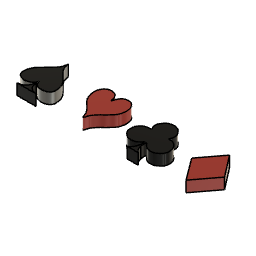
extrusion (Autodesk Fusion 360 design; units mm, degrees)
Autodesk Fusion 360 part; units mm, degrees
note: some values were not read from the file. Set by a fixed rule: which sketch regions a step uses.
sketch "Sketch1" plane through (0, 0, 0) normal (0, 0, 1) x (1, 0, 0)
  line L0 (72.8939, 22.1352) -> (57.9762, 2.4076)
  line L1 (57.9762, 2.4076) -> (72.8939, -17.6718)
  line L2 (72.8939, -17.6718) -> (88.0776, 2.4076)
  line L3 (88.0776, 2.4076) -> (72.8939, 22.1352)
  spline S0 degree 5 poles (16.5531, 7.024) (16.5732, 7.0699) (16.5975, 7.1734) (16.5852, 7.3637) (16.4741, 7.6811) (16.2192, 8.1458) (15.9092, 8.6303) (15.609, 9.0883) (15.3735, 9.4853) (15.2319, 9.8114) (15.1766, 10.0886) (15.1804, 10.3537) (15.2084, 10.645) (15.2326, 10.9866) (15.2428, 11.3775) (15.2401, 11.8016) (15.2341, 12.2351) (15.2374, 12.6541) (15.2624, 13.0428) (15.3167, 13.4004) (15.4043, 13.7352) (15.5255, 14.0605) (15.6783, 14.3894) (15.858, 14.7294) (16.0583, 15.081) (16.2727, 15.44) (16.4956, 15.8002) (16.7233, 16.1555) (16.9554, 16.5019) (17.1957, 16.8395) (17.4501, 17.1706) (17.7254, 17.4981) (18.0274, 17.8239) (18.3599, 18.1476) (18.7223, 18.4645) (19.1106, 18.7666) (19.5188, 19.0446) (19.9396, 19.2893) (20.3664, 19.4939) (20.7937, 19.6552) (21.2193, 19.7758) (21.6435, 19.8637) (22.0687, 19.9291) (22.4981, 19.9826) (22.9349, 20.0329) (23.3815, 20.0839) (23.8385, 20.1333) (24.3051, 20.1736) (24.779, 20.1952) (25.2574, 20.1876) (25.7364, 20.1421) (26.212, 20.0535) (26.6799, 19.9226) (27.1361, 19.7542) (27.5769, 19.5557) (27.9995, 19.3351) (28.4018, 19.1002) (28.7835, 18.8559) (29.1453, 18.6033) (29.4897, 18.3402) (29.8195, 18.0631) (30.1381, 17.7681) (30.4484, 17.4526) (30.753, 17.1167) (31.0531, 16.764) (31.3491, 16.4) (31.6398, 16.0304) (31.9227, 15.6599) (32.1938, 15.2907) (32.4471, 14.9207) (32.6753, 14.5431) (32.871, 14.1495) (33.0282, 13.7323) (33.1433, 13.2876) (33.2169, 12.8172) (33.2552, 12.3319) (33.2689, 11.8503) (33.2697, 11.3921) (33.2672, 10.9741) (33.2661, 10.6048) (33.263, 10.2795) (33.243, 9.975) (33.1868, 9.6587) (33.0796, 9.3006) (32.9183, 8.8831) (32.7219, 8.4143) (32.532, 7.9306) (32.3985, 7.4803) (32.3685, 7.1131) (32.4745, 6.8667) (32.7215, 6.7536) (33.0772, 6.7509) (33.4897, 6.8154) (33.9027, 6.8983) (34.2711, 6.9576) (34.5799, 6.9764) (34.8421, 6.9604) (35.0823, 6.9244) (35.3255, 6.8825) (35.582, 6.8359) (35.8511, 6.7767) (36.1269, 6.6951) (36.4039, 6.586) (36.6811, 6.4528) (36.959, 6.3023) (37.2397, 6.1425) (37.5244, 5.9781) (37.8136, 5.8092) (38.1069, 5.6327) (38.4033, 5.4433) (38.7018, 5.2353) (39.0009, 5.003) (39.2994, 4.7421) (39.5954, 4.4503) (39.887, 4.1279) (40.1718, 3.7787) (40.4468, 3.4111) (40.7088, 3.0361) (40.9548, 2.6649) (41.182, 2.3066) (41.3887, 1.9656) (41.5744, 1.6396) (41.7398, 1.3176) (41.8868, 0.9844) (42.0171, 0.6248) (42.1325, 0.2274) (42.2333, -0.2108) (42.3189, -0.682) (42.3875, -1.1721) (42.4375, -1.6639) (42.467, -2.1406) (42.4751, -2.5895) (42.462, -3.0055) (42.4295, -3.3937) (42.3799, -3.7648) (42.3152, -4.1316) (42.2364, -4.5054) (42.1426, -4.8923) (42.0305, -5.2899) (41.8959, -5.6911) (41.7348, -6.0856) (41.5448, -6.463) (41.3264, -6.8149) (41.0842, -7.1377) (40.8258, -7.4319) (40.5593, -7.7011) (40.2913, -7.9512) (40.0255, -8.1892) (39.7601, -8.4224) (39.4892, -8.6573) (39.2055, -8.8989) (38.9016, -9.1491) (38.5724, -9.4064) (38.217, -9.6647) (37.8372, -9.9149) (37.4366, -10.1471) (37.0198, -10.352) (36.5913, -10.5226) (36.154, -10.6559) (35.7095, -10.754) (35.258, -10.8217) (34.7995, -10.8654) (34.3342, -10.8917) (33.8629, -10.9056) (33.3878, -10.9091) (32.9126, -10.9007) (32.4417, -10.8768) (31.9797, -10.8328) (31.5307, -10.7639) (31.0979, -10.6662) (30.6828, -10.5379) (30.2849, -10.3798) (29.9027, -10.194) (29.5335, -9.9838) (29.1741, -9.7528) (28.8209, -9.5049) (28.4704, -9.2431) (28.1198, -8.9695) (27.7673, -8.6858) (27.413, -8.3922) (27.0589, -8.0881) (26.7098, -7.7715) (26.3734, -7.4394) (26.0589, -7.0886) (25.776, -6.717) (25.5332, -6.3247) (25.3373, -5.9148) (25.1914, -5.4946) (25.0946, -5.0759) (25.0421, -4.6716) (25.0248, -4.293) (25.0298, -3.947) (25.0402, -3.6333) (25.0354, -3.3427) (24.996, -3.0674) (24.9073, -2.8084) (24.7644, -2.5881) (24.5743, -2.448) (24.3557, -2.4249) (24.1394, -2.5245) (23.9635, -2.7139) (23.8572, -2.9499) (23.8233, -3.2046) (23.8322, -3.4791) (23.8428, -3.7855) (23.8166, -4.1369) (23.7374, -4.5318) (23.6122, -4.9537) (23.46, -5.3788) (23.3038, -5.7828) (23.1621, -6.1465) (23.0392, -6.4637) (22.9208, -6.7441) (22.7843, -7.0053) (22.606, -7.2672) (22.3706, -7.545) (22.0776, -7.8435) (21.7371, -8.1598) (21.3655, -8.486) (20.9812, -8.8109) (20.6008, -9.1229) (20.234, -9.4125) (19.8818, -9.6735) (19.5394, -9.9024) (19.1986, -10.0984) (18.8502, -10.2626) (18.4863, -10.3977) (18.103, -10.5076) (17.7001, -10.5968) (17.2808, -10.6698) (16.8518, -10.7304) (16.4222, -10.7809) (16.004, -10.8214) (15.6099, -10.8506) (15.2504, -10.8661) (14.9302, -10.8666) (14.646, -10.8518) (14.3821, -10.8247) (14.1152, -10.7896) (13.8231, -10.7492) (13.491, -10.7028) (13.119, -10.6435) (12.7173, -10.5613) (12.3015, -10.446) (11.8886, -10.2897) (11.4921, -10.09) (11.1177, -9.8523) (10.7652, -9.5878) (10.4306, -9.3099) (10.1088, -9.0317) (9.7949, -8.7629) (9.4878, -8.5064) (9.19, -8.2579) (8.9059, -8.0091) (8.6402, -7.751) (8.396, -7.4765) (8.1725, -7.1844) (7.9651, -6.8798) (7.7679, -6.5704) (7.5753, -6.2637) (7.3842, -5.9642) (7.1965, -5.6701) (7.0182, -5.3734) (6.8564, -5.0641) (6.7181, -4.7313) (6.607, -4.3668) (6.5224, -3.9667) (6.4606, -3.5312) (6.4163, -3.0638) (6.3844, -2.5713) (6.3611, -2.0629) (6.3458, -1.5505) (6.3414, -1.0471) (6.3524, -0.5655) (6.3838, -0.1167) (6.4395, 0.2919) (6.5213, 0.6577) (6.6269, 0.9852) (6.7505, 1.2851) (6.8855, 1.5702) (7.0267, 1.8529) (7.1727, 2.141) (7.3274, 2.4356) (7.4976, 2.7341) (7.6897, 3.032) (7.9081, 3.3256) (8.1516, 3.6144) (8.415, 3.9004) (8.6913, 4.186) (8.9732, 4.4726) (9.2556, 4.7593) (9.5372, 5.0403) (9.8205, 5.3069) (10.1101, 5.55) (10.4121, 5.7617) (10.7325, 5.9382) (11.0766, 6.0814) (11.4479, 6.1982) (11.8463, 6.2976) (12.2678, 6.3885) (12.7028, 6.4777) (13.1348, 6.5673) (13.5439, 6.655) (13.9132, 6.7356) (14.2338, 6.8024) (14.5101, 6.8482) (14.7676, 6.8664) (15.0424, 6.8546) (15.3618, 6.8185) (15.7281, 6.7767) (16.0992, 6.765) (16.3474, 6.8135) (16.4771, 6.8982) (16.533, 6.9782) (16.5531, 7.024) knots 0 0 0 0 0 0 0.00322581 0.00645161 0.00967742 0.01290323 0.01612903 0.01935484 0.02258065 0.02580645 0.02903226 0.03225806 0.03548387 0.03870968 0.04193548 0.04516129 0.0483871 0.0516129 0.05483871 0.05806452 0.06129032 0.06451613 0.06774194 0.07096774 0.07419355 0.07741935 0.08064516 0.08387097 0.08709677 0.09032258 0.09354839 0.09677419 0.1 0.10322581 0.10645161 0.10967742 0.11290323 0.11612903 0.11935484 0.12258065 0.12580645 0.12903226 0.13225806 0.13548387 0.13870968 0.14193548 0.14516129 0.1483871 0.1516129 0.15483871 0.15806452 0.16129032 0.16451613 0.16774194 0.17096774 0.17419355 0.17741935 0.18064516 0.18387097 0.18709677 0.19032258 0.19354839 0.19677419 0.2 0.20322581 0.20645161 0.20967742 0.21290323 0.21612903 0.21935484 0.22258065 0.22580645 0.22903226 0.23225806 0.23548387 0.23870968 0.24193548 0.24516129 0.2483871 0.2516129 0.25483871 0.25806452 0.26129032 0.26451613 0.26774194 0.27096774 0.27419355 0.27741935 0.28064516 0.28387097 0.28709677 0.29032258 0.29354839 0.29677419 0.3 0.30322581 0.30645161 0.30967742 0.31290323 0.31612903 0.31935484 0.32258065 0.32580645 0.32903226 0.33225806 0.33548387 0.33870968 0.34193548 0.34516129 0.3483871 0.3516129 0.35483871 0.35806452 0.36129032 0.36451613 0.36774194 0.37096774 0.37419355 0.37741935 0.38064516 0.38387097 0.38709677 0.39032258 0.39354839 0.39677419 0.4 0.40322581 0.40645161 0.40967742 0.41290323 0.41612903 0.41935484 0.42258065 0.42580645 0.42903226 0.43225806 0.43548387 0.43870968 0.44193548 0.44516129 0.4483871 0.4516129 0.45483871 0.45806452 0.46129032 0.46451613 0.46774194 0.47096774 0.47419355 0.47741935 0.48064516 0.48387097 0.48709677 0.49032258 0.49354839 0.49677419 0.5 0.50322581 0.50645161 0.50967742 0.51290323 0.51612903 0.51935484 0.52258065 0.52580645 0.52903226 0.53225806 0.53548387 0.53870968 0.54193548 0.54516129 0.5483871 0.5516129 0.55483871 0.55806452 0.56129032 0.56451613 0.56774194 0.57096774 0.57419355 0.57741935 0.58064516 0.58387097 0.58709677 0.59032258 0.59354839 0.59677419 0.6 0.60322581 0.60645161 0.60967742 0.61290323 0.61612903 0.61935484 0.62258065 0.62580645 0.62903226 0.63225806 0.63548387 0.63870968 0.64193548 0.64516129 0.6483871 0.6516129 0.65483871 0.65806452 0.66129032 0.66451613 0.66774194 0.67096774 0.67419355 0.67741935 0.68064516 0.68387097 0.68709677 0.69032258 0.69354839 0.69677419 0.7 0.70322581 0.70645161 0.70967742 0.71290323 0.71612903 0.71935484 0.72258065 0.72580645 0.72903226 0.73225806 0.73548387 0.73870968 0.74193548 0.74516129 0.7483871 0.7516129 0.75483871 0.75806452 0.76129032 0.76451613 0.76774194 0.77096774 0.77419355 0.77741935 0.78064516 0.78387097 0.78709677 0.79032258 0.79354839 0.79677419 0.8 0.80322581 0.80645161 0.80967742 0.81290323 0.81612903 0.81935484 0.82258065 0.82580645 0.82903226 0.83225806 0.83548387 0.83870968 0.84193548 0.84516129 0.8483871 0.8516129 0.85483871 0.85806452 0.86129032 0.86451613 0.86774194 0.87096774 0.87419355 0.87741935 0.88064516 0.88387097 0.88709677 0.89032258 0.89354839 0.89677419 0.9 0.90322581 0.90645161 0.90967742 0.91290323 0.91612903 0.91935484 0.92258065 0.92580645 0.92903226 0.93225806 0.93548387 0.93870968 0.94193548 0.94516129 0.9483871 0.9516129 0.95483871 0.95806452 0.96129032 0.96451613 0.96774194 0.97096774 0.97419355 0.97741935 0.98064516 0.98387097 0.98709677 0.99032258 0.99354839 0.99677419 1 1 1 1 1 1
  spline S1 degree 5 poles (23.2057, -6.0346) (23.2475, -6.1458) (23.3267, -6.3695) (23.4325, -6.7092) (23.5476, -7.1708) (23.6478, -7.7617) (23.7047, -8.3659) (23.719, -8.9816) (23.6925, -9.6058) (23.6286, -10.2337) (23.5321, -10.8591) (23.4082, -11.4748) (23.2619, -12.0742) (23.0969, -12.6516) (22.9155, -13.2031) (22.7172, -13.7278) (22.4996, -14.2269) (22.2602, -14.7021) (21.9965, -15.155) (21.7081, -15.5857) (21.3973, -15.9917) (21.0687, -16.3686) (20.7283, -16.7107) (20.3819, -17.0126) (20.0344, -17.2699) (19.6888, -17.4805) (19.4148, -17.6108) (19.2111, -17.6871) (19.0759, -17.7285) (19.0086, -17.7468) knots 0 0 0 0 0 0 0.04 0.08 0.12 0.16 0.2 0.24 0.28 0.32 0.36 0.4 0.44 0.48 0.52 0.56 0.6 0.64 0.68 0.72 0.76 0.8 0.84 0.88 0.92 0.96 1 1 1 1 1 1
  line L4 (19.0086, -17.7468) -> (29.1805, -17.7468)
  spline S2 degree 5 poles (25.4072, -6.0449) (25.3591, -6.0901) (25.2682, -6.1894) (25.148, -6.3647) (25.0201, -6.6512) (24.9137, -7.0959) (24.8593, -7.6215) (24.8535, -8.2166) (24.8902, -8.8616) (24.9601, -9.5264) (25.0496, -10.1677) (25.1413, -10.731) (25.2186, -11.1661) (25.2688, -11.4395) (25.2872, -11.5488) (25.2806, -11.5334) (25.2726, -11.4963) (25.2927, -11.5594) (25.3556, -11.7785) (25.4611, -12.1473) (25.6003, -12.6216) (25.7595, -13.1382) (25.9247, -13.6341) (26.0871, -14.069) (26.244, -14.4324) (26.3973, -14.7321) (26.5512, -14.988) (26.7114, -15.2238) (26.883, -15.459) (27.0692, -15.7028) (27.2717, -15.9574) (27.4916, -16.22) (27.729, -16.4857) (27.9838, -16.7497) (28.256, -17.0094) (28.5456, -17.2629) (28.791, -17.4601) (28.9828, -17.6047) (29.114, -17.6996) (29.1805, -17.7468) knots 0 0 0 0 0 0 0.028571 0.057143 0.085714 0.114286 0.142857 0.171429 0.2 0.228571 0.257143 0.285714 0.314286 0.342857 0.371429 0.4 0.428571 0.457143 0.485714 0.514286 0.542857 0.571429 0.6 0.628571 0.657143 0.685714 0.714286 0.742857 0.771429 0.8 0.828571 0.857143 0.885714 0.914286 0.942857 0.971429 1 1 1 1 1 1
  line L5 (25.4072, -6.0449) -> (23.2057, -6.0346)
  spline S3 degree 5 poles (-24.0526, 11.8543) (-24.0171, 11.9637) (-23.9443, 12.1903) (-23.8296, 12.5472) (-23.6666, 13.0371) (-23.4482, 13.6441) (-23.2171, 14.2328) (-22.9744, 14.7996) (-22.7201, 15.3444) (-22.4522, 15.8642) (-22.1673, 16.3531) (-21.8615, 16.8045) (-21.531, 17.2125) (-21.1723, 17.5731) (-20.7833, 17.886) (-20.3626, 18.1535) (-19.9093, 18.3798) (-19.4225, 18.5705) (-18.9011, 18.7319) (-18.3449, 18.8693) (-17.7563, 18.9854) (-17.1412, 19.0788) (-16.5111, 19.1419) (-15.8828, 19.1606) (-15.2745, 19.1194) (-14.7024, 19.0056) (-14.177, 18.8133) (-13.6991, 18.5487) (-13.2586, 18.2311) (-12.8409, 17.8848) (-12.4315, 17.5322) (-12.0216, 17.1879) (-11.6138, 16.8501) (-11.219, 16.5052) (-10.8511, 16.1351) (-10.5234, 15.7229) (-10.2424, 15.2598) (-10.0073, 14.748) (-9.8123, 14.1957) (-9.6498, 13.6146) (-9.5119, 13.0166) (-9.3939, 12.4099) (-9.2942, 11.7992) (-9.2132, 11.1857) (-9.1533, 10.5677) (-9.1182, 9.9412) (-9.1121, 9.2996) (-9.1397, 8.6354) (-9.205, 7.9425) (-9.3118, 7.2177) (-9.4623, 6.4628) (-9.6572, 5.6866) (-9.8951, 4.9069) (-10.1729, 4.1465) (-10.4864, 3.4291) (-10.8306, 2.7748) (-11.2006, 2.1956) (-11.5918, 1.6921) (-12.0005, 1.2473) (-12.4239, 0.8321) (-12.8593, 0.4135) (-13.3041, -0.0371) (-13.7549, -0.5364) (-14.2073, -1.0791) (-14.6559, -1.6407) (-15.0964, -2.1886) (-15.5261, -2.6908) (-15.9452, -3.1257) (-16.3582, -3.4914) (-16.775, -3.815) (-17.2072, -4.1391) (-17.6657, -4.5097) (-18.157, -4.9637) (-18.6802, -5.5145) (-19.2249, -6.1453) (-19.7751, -6.8213) (-20.3118, -7.4993) (-20.8164, -8.1386) (-21.2732, -8.7115) (-21.6729, -9.2122) (-22.0156, -9.6712) (-22.3097, -10.1427) (-22.5684, -10.6848) (-22.8065, -11.3408) (-23.0378, -12.1227) (-23.2716, -12.9869) (-23.5119, -13.84) (-23.759, -14.5675) (-24.0106, -15.0576) (-24.2632, -15.2263) (-24.5129, -15.0426) (-24.7572, -14.5521) (-24.9947, -13.8495) (-25.2251, -13.0518) (-25.4502, -12.2715) (-25.6732, -11.5904) (-25.8993, -11.0306) (-26.1349, -10.572) (-26.3861, -10.1709) (-26.658, -9.7778) (-26.9538, -9.3577) (-27.2736, -8.9023) (-27.6161, -8.4189) (-27.9792, -7.9235) (-28.3607, -7.4334) (-28.7598, -6.9574) (-29.1767, -6.4948) (-29.6122, -6.0396) (-30.0672, -5.5826) (-30.542, -5.1149) (-31.0361, -4.6311) (-31.5474, -4.1308) (-32.0729, -3.6168) (-32.6087, -3.0935) (-33.1503, -2.5653) (-33.6929, -2.0351) (-34.2314, -1.5025) (-34.7607, -0.9632) (-35.2759, -0.411) (-35.772, 0.1608) (-36.2444, 0.7576) (-36.6887, 1.3821) (-37.1008, 2.0326) (-37.4772, 2.7016) (-37.8149, 3.3782) (-38.1119, 4.0499) (-38.3676, 4.7047) (-38.5828, 5.333) (-38.76, 5.93) (-38.9039, 6.4971) (-39.0203, 7.0396) (-39.1151, 7.5651) (-39.1941, 8.0812) (-39.2619, 8.5933) (-39.3211, 9.1039) (-39.3723, 9.6143) (-39.4134, 10.126) (-39.4395, 10.6419) (-39.4424, 11.168) (-39.4126, 11.7106) (-39.3415, 12.2745) (-39.2225, 12.8612) (-39.0538, 13.4657) (-38.8382, 14.0775) (-38.5807, 14.6833) (-38.2876, 15.2692) (-37.9646, 15.8229) (-37.6148, 16.3366) (-37.2386, 16.8079) (-36.8345, 17.2376) (-36.4006, 17.6278) (-35.9353, 17.9804) (-35.4393, 18.2942) (-34.9155, 18.5652) (-34.3686, 18.7879) (-33.8039, 18.9575) (-33.2271, 19.0711) (-32.6434, 19.1301) (-32.0572, 19.1396) (-31.4721, 19.1062) (-30.8909, 19.0356) (-30.3162, 18.9311) (-29.7494, 18.7906) (-29.1922, 18.6082) (-28.6465, 18.3761) (-28.1155, 18.0867) (-27.6041, 17.735) (-27.1197, 17.3203) (-26.6712, 16.8461) (-26.2671, 16.3181) (-25.9145, 15.7437) (-25.6174, 15.1308) (-25.3753, 14.4861) (-25.1827, 13.8167) (-25.0311, 13.1349) (-24.9099, 12.4623) (-24.8072, 11.8338) (-24.7114, 11.3019) (-24.6123, 10.9405) (-24.5016, 10.8158) (-24.3735, 10.9554) (-24.2551, 11.2471) (-24.1572, 11.5339) (-24.0881, 11.7449) (-24.0526, 11.8543) knots 0 0 0 0 0 0 0.00555556 0.01111111 0.01666667 0.02222222 0.02777778 0.03333333 0.03888889 0.04444444 0.05 0.05555556 0.06111111 0.06666667 0.07222222 0.07777778 0.08333333 0.08888889 0.09444444 0.1 0.10555556 0.11111111 0.11666667 0.12222222 0.12777778 0.13333333 0.13888889 0.14444444 0.15 0.15555556 0.16111111 0.16666667 0.17222222 0.17777778 0.18333333 0.18888889 0.19444444 0.2 0.20555556 0.21111111 0.21666667 0.22222222 0.22777778 0.23333333 0.23888889 0.24444444 0.25 0.25555556 0.26111111 0.26666667 0.27222222 0.27777778 0.28333333 0.28888889 0.29444444 0.3 0.30555556 0.31111111 0.31666667 0.32222222 0.32777778 0.33333333 0.33888889 0.34444444 0.35 0.35555556 0.36111111 0.36666667 0.37222222 0.37777778 0.38333333 0.38888889 0.39444444 0.4 0.40555556 0.41111111 0.41666667 0.42222222 0.42777778 0.43333333 0.43888889 0.44444444 0.45 0.45555556 0.46111111 0.46666667 0.47222222 0.47777778 0.48333333 0.48888889 0.49444444 0.5 0.50555556 0.51111111 0.51666667 0.52222222 0.52777778 0.53333333 0.53888889 0.54444444 0.55 0.55555556 0.56111111 0.56666667 0.57222222 0.57777778 0.58333333 0.58888889 0.59444444 0.6 0.60555556 0.61111111 0.61666667 0.62222222 0.62777778 0.63333333 0.63888889 0.64444444 0.65 0.65555556 0.66111111 0.66666667 0.67222222 0.67777778 0.68333333 0.68888889 0.69444444 0.7 0.70555556 0.71111111 0.71666667 0.72222222 0.72777778 0.73333333 0.73888889 0.74444444 0.75 0.75555556 0.76111111 0.76666667 0.77222222 0.77777778 0.78333333 0.78888889 0.79444444 0.8 0.80555556 0.81111111 0.81666667 0.82222222 0.82777778 0.83333333 0.83888889 0.84444444 0.85 0.85555556 0.86111111 0.86666667 0.87222222 0.87777778 0.88333333 0.88888889 0.89444444 0.9 0.90555556 0.91111111 0.91666667 0.92222222 0.92777778 0.93333333 0.93888889 0.94444444 0.95 0.95555556 0.96111111 0.96666667 0.97222222 0.97777778 0.98333333 0.98888889 0.99444444 1 1 1 1 1 1
  spline S4 degree 5 poles (-73.0409, 20.47) (-73.074, 20.3206) (-73.1394, 20.0245) (-73.235, 19.5893) (-73.3577, 19.0265) (-73.5042, 18.3517) (-73.6475, 17.7039) (-73.7945, 17.0799) (-73.9575, 16.4739) (-74.1535, 15.8779) (-74.4, 15.2835) (-74.7117, 14.6832) (-75.0965, 14.0724) (-75.5518, 13.4507) (-76.0672, 12.8209) (-76.6275, 12.1879) (-77.2153, 11.5567) (-77.8143, 10.9321) (-78.4121, 10.3163) (-79.0008, 9.7096) (-79.5763, 9.1112) (-80.1376, 8.5196) (-80.686, 7.9336) (-81.2246, 7.3533) (-81.7578, 6.7802) (-82.2897, 6.2164) (-82.8231, 5.6635) (-83.3584, 5.1216) (-83.8921, 4.5881) (-84.416, 4.0567) (-84.919, 3.5188) (-85.3899, 2.9655) (-85.8199, 2.389) (-86.2048, 1.7842) (-86.5476, 1.1505) (-86.8556, 0.4901) (-87.1369, -0.1938) (-87.3984, -0.8988) (-87.642, -1.6244) (-87.8629, -2.3736) (-88.0517, -3.1502) (-88.1962, -3.956) (-88.2831, -4.7887) (-88.3003, -5.6396) (-88.2388, -6.4904) (-88.0926, -7.3173) (-87.859, -8.0955) (-87.5388, -8.8035) (-87.1362, -9.4273) (-86.659, -9.9659) (-86.1178, -10.4302) (-85.5239, -10.8356) (-84.8876, -11.197) (-84.2164, -11.5233) (-83.513, -11.81) (-82.7767, -12.0432) (-82.0064, -12.2049) (-81.2029, -12.2788) (-80.3712, -12.2549) (-79.5242, -12.1367) (-78.6807, -11.9391) (-77.8622, -11.6826) (-77.0901, -11.3887) (-76.3821, -11.0746) (-75.7496, -10.7477) (-75.1946, -10.4023) (-74.7133, -10.0244) (-74.2987, -9.5958) (-73.943, -9.0993) (-73.6407, -8.5227) (-73.3885, -7.859) (-73.2256, -7.2556) (-73.1249, -6.7618) (-73.0673, -6.4143) (-73.0409, -6.2359) knots 0 0 0 0 0 0 0.01428571 0.02857143 0.04285714 0.05714286 0.07142857 0.08571429 0.1 0.11428571 0.12857143 0.14285714 0.15714286 0.17142857 0.18571429 0.2 0.21428571 0.22857143 0.24285714 0.25714286 0.27142857 0.28571429 0.3 0.31428571 0.32857143 0.34285714 0.35714286 0.37142857 0.38571429 0.4 0.41428571 0.42857143 0.44285714 0.45714286 0.47142857 0.48571429 0.5 0.51428571 0.52857143 0.54285714 0.55714286 0.57142857 0.58571429 0.6 0.61428571 0.62857143 0.64285714 0.65714286 0.67142857 0.68571429 0.7 0.71428571 0.72857143 0.74285714 0.75714286 0.77142857 0.78571429 0.8 0.81428571 0.82857143 0.84285714 0.85714286 0.87142857 0.88571429 0.9 0.91428571 0.92857143 0.94285714 0.95714286 0.97142857 0.98571429 1 1 1 1 1 1
  spline S5 degree 5 poles (-73.0409, 20.47) (-73.0112, 20.3318) (-72.9527, 20.0576) (-72.868, 19.6527) (-72.7609, 19.126) (-72.6357, 18.4884) (-72.5148, 17.8694) (-72.39, 17.2641) (-72.2469, 16.6645) (-72.0659, 16.0592) (-71.8262, 15.4367) (-71.5097, 14.787) (-71.1046, 14.1045) (-70.6102, 13.3907) (-70.0354, 12.6527) (-69.3956, 11.9013) (-68.7097, 11.1486) (-67.9973, 10.4061) (-67.2763, 9.6824) (-66.5591, 8.981) (-65.8512, 8.2988) (-65.1535, 7.6285) (-64.464, 6.9601) (-63.7801, 6.2828) (-63.1005, 5.5872) (-62.4272, 4.8665) (-61.7678, 4.1193) (-61.1351, 3.349) (-60.5444, 2.5623) (-60.011, 1.7674) (-59.5475, 0.9724) (-59.1615, 0.184) (-58.8532, -0.5949) (-58.6127, -1.3659) (-58.4245, -2.1339) (-58.272, -2.9049) (-58.1419, -3.6842) (-58.0285, -4.475) (-57.939, -5.2756) (-57.8931, -6.0795) (-57.9161, -6.8764) (-58.0335, -7.6535) (-58.2648, -8.3962) (-58.6177, -9.0895) (-59.0822, -9.719) (-59.6371, -10.2721) (-60.255, -10.7399) (-60.9086, -11.1182) (-61.5756, -11.4093) (-62.2455, -11.6234) (-62.9176, -11.7761) (-63.5965, -11.8838) (-64.2891, -11.9599) (-65.0007, -12.0112) (-65.7317, -12.0332) (-66.4771, -12.0149) (-67.2274, -11.9426) (-67.9682, -11.8053) (-68.6806, -11.598) (-69.3411, -11.3279) (-69.9264, -11.0103) (-70.4187, -10.6635) (-70.8112, -10.3051) (-71.1147, -9.9456) (-71.3585, -9.5867) (-71.5763, -9.2247) (-71.7953, -8.8537) (-72.0229, -8.4688) (-72.254, -8.0664) (-72.4779, -7.6437) (-72.6865, -7.1991) (-72.8384, -6.8253) (-72.9432, -6.5347) (-73.009, -6.3363) (-73.0409, -6.2359) knots 0 0 0 0 0 0 0.01428571 0.02857143 0.04285714 0.05714286 0.07142857 0.08571429 0.1 0.11428571 0.12857143 0.14285714 0.15714286 0.17142857 0.18571429 0.2 0.21428571 0.22857143 0.24285714 0.25714286 0.27142857 0.28571429 0.3 0.31428571 0.32857143 0.34285714 0.35714286 0.37142857 0.38571429 0.4 0.41428571 0.42857143 0.44285714 0.45714286 0.47142857 0.48571429 0.5 0.51428571 0.52857143 0.54285714 0.55714286 0.57142857 0.58571429 0.6 0.61428571 0.62857143 0.64285714 0.65714286 0.67142857 0.68571429 0.7 0.71428571 0.72857143 0.74285714 0.75714286 0.77142857 0.78571429 0.8 0.81428571 0.82857143 0.84285714 0.85714286 0.87142857 0.88571429 0.9 0.91428571 0.92857143 0.94285714 0.95714286 0.97142857 0.98571429 1 1 1 1 1 1
  spline S6 degree 5 poles (-73.0214, -9.058) (-73.052, -9.161) (-73.1115, -9.3631) (-73.1957, -9.6544) (-73.2979, -10.0192) (-73.409, -10.4363) (-73.5046, -10.8164) (-73.5873, -11.1634) (-73.6611, -11.4842) (-73.7327, -11.7896) (-73.8097, -12.0916) (-73.9008, -12.401) (-74.0142, -12.7254) (-74.1575, -13.0661) (-74.336, -13.4203) (-74.5521, -13.7824) (-74.8041, -14.1457) (-75.0847, -14.5039) (-75.3819, -14.8521) (-75.6823, -15.1863) (-75.9749, -15.5038) (-76.2534, -15.8025) (-76.5207, -16.0816) (-76.7893, -16.3409) (-77.0768, -16.5806) (-77.4031, -16.8014) (-77.7867, -17.0041) (-78.2412, -17.1894) (-78.7758, -17.3578) (-79.396, -17.5099) (-80.1048, -17.6459) (-80.7436, -17.7421) (-81.263, -17.8072) (-81.6272, -17.8474) (-81.8137, -17.8668) knots 0 0 0 0 0 0 0.033333 0.066667 0.1 0.133333 0.166667 0.2 0.233333 0.266667 0.3 0.333333 0.366667 0.4 0.433333 0.466667 0.5 0.533333 0.566667 0.6 0.633333 0.666667 0.7 0.733333 0.766667 0.8 0.833333 0.866667 0.9 0.933333 0.966667 1 1 1 1 1 1
  line L6 (-81.8137, -17.8668) -> (-64.3804, -17.8668)
  spline S7 degree 5 poles (-64.3804, -17.8668) (-64.5168, -17.8472) (-64.7844, -17.8076) (-65.1703, -17.7474) (-65.6536, -17.6651) (-66.206, -17.5586) (-66.7078, -17.4478) (-67.1617, -17.3307) (-67.5724, -17.2044) (-67.9479, -17.0645) (-68.2991, -16.9049) (-68.6378, -16.7198) (-68.9736, -16.5053) (-69.3123, -16.2615) (-69.6522, -15.994) (-69.985, -15.7136) (-70.2999, -15.4312) (-70.587, -15.1549) (-70.8398, -14.8859) (-71.0599, -14.6145) (-71.2547, -14.3235) (-71.4342, -13.9943) (-71.6082, -13.6126) (-71.7827, -13.1739) (-71.9591, -12.6862) (-72.1353, -12.165) (-72.3072, -11.6304) (-72.4698, -11.1033) (-72.6184, -10.6026) (-72.7497, -10.141) (-72.8619, -9.7257) (-72.9358, -9.4333) (-72.9821, -9.2368) (-73.0089, -9.1159) (-73.0214, -9.058) knots 0 0 0 0 0 0 0.033333 0.066667 0.1 0.133333 0.166667 0.2 0.233333 0.266667 0.3 0.333333 0.366667 0.4 0.433333 0.466667 0.5 0.533333 0.566667 0.6 0.633333 0.666667 0.7 0.733333 0.766667 0.8 0.833333 0.866667 0.9 0.933333 0.966667 1 1 1 1 1 1
  point P0 (15.4343, 9.3971)
  point P1 (15.2026, 10.5941)
  point P2 (15.2413, 12.6019)
  point P3 (15.6154, 14.2471)
  point P4 (16.6763, 16.0796)
  point P5 (18.123, 17.9121)
  point P6 (20.5342, 19.5517)
  point P7 (22.9454, 20.0339)
  point P8 (25.7423, 20.1304)
  point P9 (28.4428, 19.0695)
  point P10 (30.3718, 17.5263)
  point P11 (32.1078, 15.4045)
  point P12 (33.1688, 13.0897)
  point P13 (33.2652, 10.5821)
  point P14 (32.9759, 9.039)
  point P15 (32.4936, 6.9171)
  point P16 (34.0368, 6.9171)
  point P17 (35.1185, 6.9171)
  point P18 (36.0318, 6.7197)
  point P19 (37.1452, 6.1958)
  point P20 (38.4223, 5.4262)
  point P21 (39.9451, 4.0509)
  point P22 (41.3532, 2.0206)
  point P23 (42.1007, 0.3229)
  point P24 (42.4698, -2.4822)
  point P25 (42.2483, -4.4384)
  point P26 (41.5102, -6.5053)
  point P27 (40.2553, -7.9816)
  point P28 (38.9265, -9.1258)
  point P29 (36.7489, -10.4545)
  point P30 (34.0915, -10.8974)
  point P31 (31.3233, -10.7129)
  point P32 (29.1826, -9.7532)
  point P33 (27.1526, -8.1662)
  point P34 (25.4072, -6.0449)
  point P35 (25.0303, -4.0035)
  point P36 (24.93, -2.9006)
  point P37 (24.4287, -2.4494)
  point P38 (23.9023, -2.8756)
  point P39 (23.8271, -3.9283)
  point P40 (23.2057, -6.0346)
  point P41 (22.6128, -7.2434)
  point P42 (20.7305, -9.0151)
  point P43 (18.8112, -10.27)
  point P44 (16.6763, -10.7498)
  point P45 (14.862, -10.8605)
  point P46 (13.8285, -10.7498)
  point P47 (11.8724, -10.27)
  point P48 (9.9162, -8.8674)
  point P49 (8.5012, -7.5895)
  point P50 (7.5171, -6.1731)
  point P51 (6.742, -4.7705)
  point P52 (6.3729, -2.2976)
  point P53 (6.4837, 0.4705)
  point P54 (7.0004, 1.7992)
  point P55 (7.7386, 3.091)
  point P56 (9.0304, 4.5305)
  point P57 (10.4698, 5.7854)
  point P58 (12.3891, 6.4128)
  point P59 (14.3159, 6.8137)
  point P60 (15.4058, 6.8137)
  point P61 (23.7009, -9.293)
  point P62 (23.0697, -12.7196)
  point P63 (21.9243, -15.2535)
  point P64 (20.397, -16.989)
  point P65 (24.9389, -9.293)
  point P66 (25.2823, -11.5288)
  point P67 (25.2823, -11.5288)
  point P68 (25.8457, -13.3913)
  point P69 (26.6869, -15.1843)
  point P70 (27.6332, -16.376)
  point P71 (-22.9285, 14.8895)
  point P72 (-21.5795, 17.1377)
  point P73 (-19.8933, 18.3743)
  point P74 (-17.3078, 19.0488)
  point P75 (-14.3544, 18.8655)
  point P76 (-12.3616, 17.475)
  point P77 (-10.6754, 15.9012)
  point P78 (-9.6193, 13.4635)
  point P79 (-9.1442, 10.3416)
  point P80 (-9.4835, 6.4128)
  point P81 (-11.316, 2.0616)
  point P82 (-13.4878, -0.2459)
  point P83 (-15.931, -3.0964)
  point P84 (-18.035, -4.861)
  point P85 (-21.3719, -8.8358)
  point P86 (-22.9141, -11.7191)
  point P87 (-24.2552, -15.1389)
  point P88 (-25.4622, -12.2555)
  point P89 (-26.5864, -9.8833)
  point P90 (-28.1474, -7.7115)
  point P91 (-30.3871, -5.2682)
  point P92 (-33.509, -2.2141)
  point P93 (-36.631, 1.3151)
  point P94 (-38.5516, 5.2582)
  point P95 (-39.1625, 7.8847)
  point P96 (-39.4068, 10.0837)
  point P97 (-39.2846, 12.527)
  point P98 (-38.063, 15.6421)
  point P99 (-36.1084, 17.8411)
  point P100 (-33.5429, 19.0016)
  point P101 (-30.7332, 19.0016)
  point P102 (-28.0456, 18.0243)
  point P103 (-25.7856, 15.4589)
  point P104 (-24.8083, 11.8543)
  point P105 (-24.501, 10.8812)
  point P106 (-73.7493, 17.2823)
  point P107 (-74.741, 14.6613)
  point P108 (-77.4329, 11.3319)
  point P109 (-80.6206, 8.0025)
  point P110 (-83.3833, 5.0981)
  point P111 (-85.7918, 2.4063)
  point P112 (-87.3502, -0.7814)
  point P113 (-88.2711, -4.89)
  point P114 (-87.3502, -9.0695)
  point P115 (-84.7292, -11.2655)
  point P116 (-80.904, -12.2572)
  point P117 (-76.512, -11.1238)
  point P118 (-74.2452, -9.4945)
  point P119 (-72.4358, 17.496)
  point P120 (-71.3856, 14.5956)
  point P121 (-67.4352, 9.8451)
  point P122 (-62.7847, 5.2446)
  point P123 (-59.1843, 0.1941)
  point P124 (-58.0842, -4.1064)
  point P125 (-58.2842, -8.3569)
  point P126 (-61.0345, -11.1572)
  point P127 (-64.3349, -11.9573)
  point P128 (-68.0853, -11.7573)
  point P129 (-70.6856, -10.4071)
  point P130 (-71.5857, -9.207)
  point P131 (-72.3358, -7.9068)
  point P132 (-73.5823, -11.145)
  point P133 (-73.9058, -12.4031)
  point P134 (-74.6966, -13.9847)
  point P135 (-76.1344, -15.6741)
  point P136 (-77.4644, -16.8244)
  point P137 (-67.5076, -17.2198)
  point P138 (-69.1252, -16.393)
  point P139 (-70.6348, -15.099)
  point P140 (-71.5335, -13.769)
  point P141 (-72.4984, -11.0035)
  constraint parallel L0 L2
  constraint horizontal L4
  constraint coincident P67 P66
  constraint coincident P34 S2.start
  constraint coincident P40 S1.start
  constraint horizontal L6
extrude "Extrude1" add sketch "Sketch1" along normal blind 10 makes body 1 at (-76.0026, -17.8668, 3.3333) makes body 2 at (-72.5678, 4.8153, 0) makes body 3 at (-21.3699, -8.8333, 5.0181) makes body 4 at (28.4782, -9.2461, 4.1985) makes body 5 at (72.9826, -4.2855, 0)
